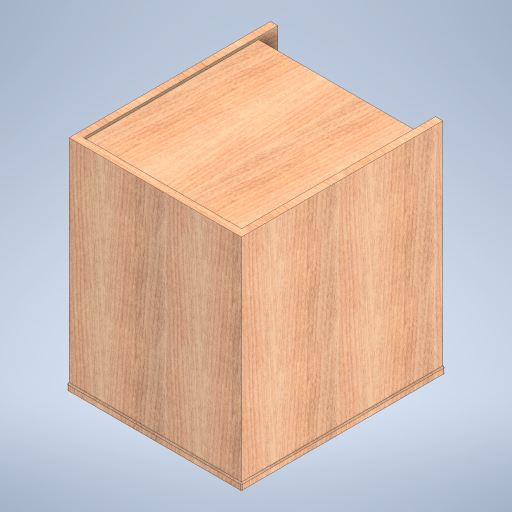
# Autodesk Inventor part: SmallDrawer
Saved by Autodesk Inventor 2023 (Build 270158000, 158)
## iProperties
Created: 2022-09-18
Part Number: SmallDrawer
Material: Wood (Birch)
Document SubType Name: Modeling
Designer: mliu-23
Density: 0.55 g/cm^3
Appearance: Birch - Natural Polished
Author: mliu-23
Autodesk Inventor part; units mm, degrees
ref_plane "YZ Plane" through (0, 0, 0) normal (1, 0, 0) x (0, 1, 0)
ref_plane "XZ Plane" through (0, 0, 0) normal (0, 1, 0) x (-1, 0, 0)
ref_plane "XY Plane" through (0, 0, 0) normal (0, 0, 1) x (1, 0, 0)
sketch "Sketch1" plane through (0, 0, 0) normal (0, 1, 0) x (-1, 0, 0)
  line L0 (0, 0) -> (-457.2, 0)
  line L1 (-457.2, 0) -> (-457.2, 533.4)
  line L2 (-457.2, 533.4) -> (0, 533.4)
  line L3 (0, 533.4) -> (0, 0)
  dimension "d0" = 457.2
  dimension "d1" = 533.4
  constraints: 8 end point, 2 parallel, 1 horizontal, 1 perpendicular
  measures "d0" distance of L1.end L2.end
  measures "d1" distance of L0.end L1.end
extrude "Extrusion1" add sketch "Sketch1" along normal blind 19.05
sketch "Sketch2" plane through (0, 19.05, 0) normal (0, 1, 0) x (1, 0, 0)
  line L0 (0, -533.4) -> (457.2, -533.4) projected
  line L1 (457.2, -533.4) -> (457.2, 0) projected
  line L2 (457.2, 0) -> (0, 0) projected
  line L3 (0, 0) -> (0, -533.4) projected
  line L4 (3.175, -530.225) -> (454.025, -530.225)
  line L5 (454.025, -530.225) -> (454.025, -3.175)
  line L6 (454.025, -3.175) -> (3.175, -3.175)
  line L7 (3.175, -3.175) -> (3.175, -530.225)
  dimension "d4" = 3.175
  constraints: 8 end point, 3 other
  measures "d4" distance between parallel lines of L3 L7
extrude "Extrusion2" add sketch "Sketch2" along normal blind 555.625 contours L7 L6 L5 L4
sketch "Sketch3" plane through (454.025, 19.05, 3.175) normal (0, 0, -1) x (-1, 0, 0)
  line L0 (454.025, 0) -> (-3.175, 0) projected
  line L1 (450.85, 555.625) -> (0, 555.625) projected
  line L2 (431.8, 0) -> (19.05, 0)
  line L3 (19.05, 0) -> (19.05, 555.625)
  line L4 (19.05, 555.625) -> (431.8, 555.625)
  line L5 (431.8, 555.625) -> (431.8, 0)
  line L6 (450.85, 0) -> (450.85, 555.625) projected
  line L7 (0, 0) -> (0, 555.625) projected
  point P0 (454.025, -19.05)
  point P1 (19.05, 0)
  dimension "d7" = 19.05
  dimension "d8" = 19.05
  constraints: 8 end point, 2 parallel, 2 point on line, 1 horizontal, 1 perpendicular
  measures "d7" distance between parallel lines of L5 L6
  measures "d8" distance between parallel lines of L7 L3
extrude "Extrusion3" cut sketch "Sketch3" against normal blind 50.8 contours L0 L3 L1 L5
sketch "Sketch4" plane through (454.025, 19.05, 53.975) normal (0, 0, -1) x (-1, 0, 0)
  line L0 (19.05, 0) -> (19.05, 555.625) projected
  line L1 (431.8, 555.625) -> (19.05, 555.625)
  line L2 (19.05, 555.625) -> (19.05, 549.275)
  line L3 (19.05, 549.275) -> (431.8, 549.275)
  line L4 (431.8, 549.275) -> (431.8, 555.625)
  point P0 (454.025, -19.05)
  dimension "d11" = 6.35
  constraints: 8 end point, 2 parallel, 1 horizontal, 1 perpendicular, 1 point on line
  measures "d11" distance between parallel lines of L1 L3
extrude "Extrusion4" cut sketch "Sketch4" against normal blind 457.2
sketch "Sketch5" plane through (454.025, 19.05, 53.975) normal (0, 0, -1) x (-1, 0, 0)
  line L0 (412.75, 193.675) -> (38.1, 193.675)
  line L1 (38.1, 193.675) -> (38.1, 498.475)
  line L2 (38.1, 498.475) -> (412.75, 498.475)
  line L3 (412.75, 498.475) -> (412.75, 193.675)
  line L4 (412.75, 12.7) -> (38.1, 12.7)
  line L5 (38.1, 12.7) -> (38.1, 180.975)
  line L6 (38.1, 180.975) -> (412.75, 180.975)
  line L7 (412.75, 180.975) -> (412.75, 12.7)
  line L8 (431.8, 555.625) -> (431.8, 0) projected
  line L9 (19.05, 0) -> (19.05, 555.625) projected
  line L10 (431.8, 549.275) -> (19.05, 549.275) projected
  line L11 (-3.175, 0) -> (454.025, 0) projected
  point P0 (454.025, -19.05)
  point P1 (38.1, 96.8375)
  point P2 (225.425, 549.275)
  dimension "d14" = 19.05
  dimension "d15" = 19.05
  dimension "d16" = 19.05
  dimension "d17" = 19.05
  dimension "d18" = 50.8
  dimension "d19" = 304.8
  dimension "d20" = 12.7
  dimension "d21" = 12.7
  constraints: 16 end point, 4 parallel, 2 horizontal, 2 midpoint, 2 perpendicular
  measures "d14" distance between parallel lines of L8 L7
  measures "d15" distance from line of L9 point (38.1, 96.837)
  measures "d16" distance between parallel lines of L9 L1
  measures "d17" distance between parallel lines of L8 L3
  measures "d18" distance from line of point (225.425, 549.275) L2
  measures "d19" distance of L2.end L0.start
  measures "d20" distance between parallel lines of L0 L6
  measures "d21" distance between parallel lines of L11 L4
extrude "Extrusion5" add sketch "Sketch5" along normal blind 38.1 contours L0 L1 L2 L3 | L4 L5 L6 L7
sketch "Sketch6" plane through (415.925, 31.75, 53.975) normal (1, 0, 0) x (0, 0, -1)
  line L0 (0, 168.275) -> (0, 0) projected
  line L1 (0, 168.275) -> (38.1, 168.275) projected
  line L2 (38.1, 0) -> (38.1, 168.275) projected
  line L3 (0, 0) -> (38.1, 0) projected
  line L4 (0, 485.775) -> (0, 180.975) projected
  line L5 (0, 485.775) -> (38.1, 485.775) projected
  line L6 (38.1, 180.975) -> (38.1, 485.775) projected
  line L7 (0, 180.975) -> (38.1, 180.975) projected
  line L8 (38.1, 0) -> (0, 25.4)
  line L9 (38.1, 168.275) -> (0, 142.875)
  line L10 (38.1, 180.975) -> (0, 206.375)
  line L11 (38.1, 485.775) -> (0, 460.375)
  line L12 (0, 536.575) -> (0, -12.7) projected
  point P0 (53.975, -31.75)
  point P1 (38.1, 0)
  dimension "d24" = 25.4
  constraints: 8 end point, 3 equal length, 3 point on line, 2 other
  measures "d24" distance of L8.end L0.end
extrude "Extrusion6" cut sketch "Sketch6" against normal up to surface (374.65 mm away) contours L1 L9 L0 | L8 L3 L0 | L5 L11 L4 | L10 L7 L4
fillet "Fillet1" radius 3.175 8 edges at (457.2, 0, 266.7) (457.2, 19.05, 266.7) (228.6, 0, 0) (228.6, 19.05, 0) (0, 0, 266.7) (0, 19.05, 266.7) (228.6, 19.05, 533.4) (228.6, 0, 533.4)
fillet "Fillet2" radius 3.175 12 edges at (457.2, 9.525, 0) (456.2701, 18.1201, 0.9299) (456.2701, 0.9299, 0.9299) (456.2701, 18.1201, 532.4701) (456.2701, 0.9299, 532.4701) (457.2, 9.525, 533.4) (0.9299, 18.1201, 0.9299) (0.9299, 0.9299, 0.9299) (0, 9.525, 0) (0.9299, 18.1201, 532.4701) (0.9299, 0.9299, 532.4701) (0, 9.525, 533.4)
fillet "Fillet3" radius 9.525 4 edges at (228.6, 31.75, 15.875) (228.6, 200.025, 15.875) (228.6, 212.725, 15.875) (228.6, 517.525, 15.875)
body "Solid1"
